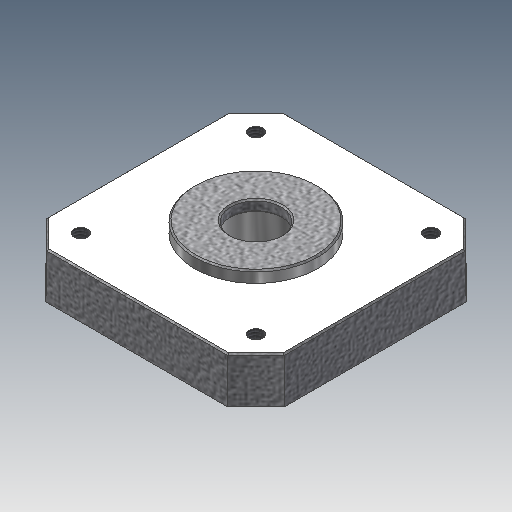
# Autodesk Inventor part: Nema 17 Top Cap
Saved by Autodesk Inventor 2020.2 (Build 242310000, 310)
## iProperties
Created: 2020-01-17
Part Number: Nema 17 Top Cap
Material: Aluminum 6061
Document SubType Name: Modeling
Designer: james
Density: 2.7 g/cm^3
Appearance: Aluminum Cast
Mass: 23.5583 g
Surface Area: 66.2945 cm^2
Volume: 8.7253 cm^3
Author: james
Autodesk Inventor part; units mm, degrees
ref_plane "YZ Plane" through (0, 0, 0) normal (1, 0, 0) x (0, 1, 0)
ref_plane "XZ Plane" through (0, 0, 0) normal (0, 1, 0) x (-1, 0, 0)
ref_plane "XY Plane" through (0, 0, 0) normal (0, 0, 1) x (1, 0, 0)
sketch "Sketch11" plane through (0, 0, 0) normal (0, 1, 0) x (-1, 0, 0)
  line L0 (-16, 21) -> (16, 21)
  line L1 (21, 16) -> (21, -16)
  line L2 (16, -21) -> (-16, -21)
  line L3 (-21, -16) -> (-21, 16)
  line L4 (-21, 21) -> (21, -21) construction
  line L5 (21, 21) -> (-21, -21) construction
  line L6 (21, -16) -> (16, -21)
  line L7 (-16, -21) -> (-21, -16)
  line L8 (-21, 16) -> (-16, 21)
  line L9 (16, 21) -> (21, 16)
  point P0 (0, 0)
  dimension "d82" = 42
  dimension "d83" = 5
  dimension "d84" = 5
  dimension "d85" = 5
  dimension "d86" = 5
  dimension "d87" = 5
  dimension "d88" = 5
  dimension "d89" = 5
  dimension "d90" = 5
  constraints: 20 end point, 8 point on line, 2 midpoint, 2 parallel, 2 perpendicular, 1 horizontal
  measures "d82" distance between parallel lines of L0 L2
  measures "d83" distance of L1.end L4.end
  measures "d84" distance of L2.start L4.end
  measures "d85" distance of L2.end L5.end
  measures "d86" distance of L3.start L5.end
  measures "d87" distance of L3.end L4.start
  measures "d88" distance of L0.start L4.start
  measures "d89" distance of L0.end L5.start
  measures "d90" distance of L1.start L5.start
extrude "Extrusion7" add sketch "Sketch11" against normal blind 8 draft 1
sketch "Sketch12" plane through (0, 0, 0) normal (0, 1, 0) x (1, 0, 0)
  circle A0 centre (0, 0) radius 10.9
  dimension "d93" = 21.8
  constraints: 1 centre point, 1 coincident
  measures "d93" diameter of A0
extrude "Extrusion8" add sketch "Sketch12" along normal blind 2
sketch "Sketch13" plane through (0, -8, 0) normal (0, -1, 0) x (1, 0, 0)
  circle A0 centre (0, 0) radius 13
  line L0 (-8.0772, 19.5) -> (8.0772, 19.5)
  line L1 (8.0772, 19.5) -> (19.5, 8.0772)
  line L2 (19.5, 8.0772) -> (19.5, -8.0772)
  line L3 (19.5, -8.0772) -> (8.0772, -19.5)
  line L4 (8.0772, -19.5) -> (-8.0772, -19.5)
  line L5 (-8.0772, -19.5) -> (-19.5, -8.0772)
  line L6 (-19.5, -8.0772) -> (-19.5, 8.0772)
  line L7 (-19.5, 8.0772) -> (-8.0772, 19.5)
  dimension "d96" = 26
  dimension "d97" = 39
  constraints: 16 end point, 2 coincident, 1 centre point, 1 vertical, 17 other
  measures "d96" diameter of A0
  measures "d97" distance between parallel lines of L2 L6
extrude "Extrusion9" cut sketch "Sketch13" against normal blind 6
sketch "Sketch14" plane through (0, -8, 0) normal (0, -1, 0) x (1, 0, 0)
  circle A0 centre (0, 0) radius 13 projected
extrude "Extrusion10" add sketch "Sketch14" along normal blind 1
sketch "Sketch15" plane through (0, -9, 0) normal (0, -1, 0) x (1, 0, 0)
  circle A0 centre (0, 0) radius 8
  dimension "d102" = 16
  constraints: 1 centre point, 1 coincident
  measures "d102" diameter of A0
extrude "Extrusion11" cut sketch "Sketch15" against normal blind 8.25
sketch "Sketch16" plane through (0, 2, 0) normal (0, 1, 0) x (1, 0, 0)
  point P0 (0, 0)
  point P1 (0, 0)
  constraints: 1 coincident
hole "Hole5" at (0, 2, 0) direction (0, -1, 0) diameter 9 end through all
sketch "Sketch17" plane through (0, -0.75, 0) normal (0, -1, 0) x (1, 0, 0)
  circle A0 centre (0, 0) radius 6
  dimension "d112" = 12
  constraints: 1 centre point, 1 coincident
  measures "d112" diameter of A0
extrude "Extrusion12" cut sketch "Sketch17" against normal blind 0.75
sketch "Sketch18" plane through (0, 0, 0) normal (0, 1, 0) x (1, 0, 0)
  line L0 (-15.5, 15.5) -> (15.5, 15.5) construction
  line L1 (15.5, 15.5) -> (15.5, -15.5) construction
  line L2 (15.5, -15.5) -> (-15.5, -15.5) construction
  line L3 (-15.5, -15.5) -> (-15.5, 15.5) construction
  line L4 (-15.5, 15.5) -> (15.5, -15.5) construction
  line L5 (15.5, 15.5) -> (-15.5, -15.5) construction
  point P0 (0, 0)
  point P1 (0, 0)
  dimension "d115" = 31
  dimension "d124" = 31
  constraints: 12 end point, 2 midpoint, 1 coincident, 1 horizontal, 1 vertical
  measures "d115" distance of L0.start L0.end
  measures "d124" distance of L2.end L0.start
hole "Hole6" at (-15.5, 0, -15.5) at (15.5, 0, -15.5) at (15.5, 0, 15.5) at (-15.5, 0, 15.5) direction (0, -1, 0) diameter 2.459 end through all thread size "M3x0.5" class "6H" standard "ISO Metric profile"
chamfer "Chamfer1" distance 0.25 distance2 1 1 edges at (-8, -9, 0) measured on face at (11.1299, -9, -1.6752)
chamfer "Chamfer2" distance 0.25 angle 45 12 edges at (-13, -9, 0) (0, 0, -4.5) (0, 2, -4.5) (-10.9, 2, 0) (-21, 0, 0) (-18.5, 0, 18.5) (0, 0, 21) (18.5, 0, 18.5) (21, 0, 0) (18.5, 0, -18.5) (0, 0, -21) (-18.5, 0, -18.5)
chamfer "Chamfer3" distance 1 angle 45 8 edges at (-13.7886, -2, -13.7886) (-19.5, -2, 0) (-13.7886, -2, 13.7886) (0, -2, 19.5) (13.7886, -2, 13.7886) (19.5, -2, 0) (13.7886, -2, -13.7886) (0, -2, -19.5)
equation "\"d84\" = d83"
equation "\"d85\" = d83"
equation "\"d86\" = d85"
equation "\"d87\" = d83"
equation "\"d88\" = d87"
equation "\"d89\" = d83"
equation "\"d90\" = d89"
body "Solid6"
